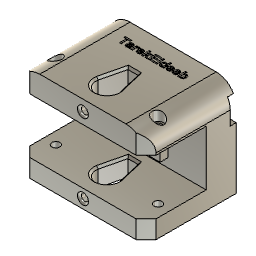
pltr_base_elegoo (Autodesk Fusion 360 design; units mm, degrees)
Autodesk Fusion 360 part; units mm, degrees
sketch "Top" plane through (0, 0, 0) normal (0, 0, 1) x (1, 0, 0)
  line L0 (0, 0) -> (-63, 0)
  line L1 (-63, 0) -> (-63, 35)
  line L2 (-63, 35) -> (0, 35)
  line L3 (0, 35) -> (0, 0)
  line L4 (-63, 12) -> (0, 12)
  line L5 (-6, 35) -> (-6, 0)
  line L6 (-57, 0) -> (-57, 35)
  line L7 (-31.5, 35) -> (-31.5, 0)
  line L8 (-63, 25) -> (0, 25)
  circle A0 centre (-31.5, 12) radius 5.5
  line L9 (-34, 25) -> (-29, 25)
  line L10 (-34, 25) -> (-36.91568, 12.95938)
  line L11 (-29, 25) -> (-26.15564, 13.299162)
  circle A1 centre (-6, 12) radius 3
  circle A2 centre (-6, 12) radius 2
  circle A3 centre (-57, 12) radius 3
  circle A4 centre (-57, 12) radius 2
  line L12 (-63, 35) -> (0, 35)
  line L13 (0, 35) -> (0, 45)
  line L14 (0, 45) -> (-63, 45)
  line L15 (-63, 45) -> (-63, 35)
  line L16 (-3.293913, 9.66023) -> (-2.620656, 13.173655)
  line L17 (-2.620656, 13.173655) -> (-5.326743, 15.513426)
  line L18 (-5.326743, 15.513426) -> (-8.706088, 14.339771)
  line L19 (-8.706088, 14.339771) -> (-9.379345, 10.826345)
  line L20 (-9.379345, 10.826345) -> (-6.673257, 8.486574)
  line L21 (-6.673257, 8.486574) -> (-3.293913, 9.66023)
  line L22 (-57.673257, 15.513426) -> (-54.293912, 14.339771)
  line L23 (-54.293912, 14.339771) -> (-53.620655, 10.826345)
  line L24 (-53.620655, 10.826345) -> (-56.326743, 8.486574)
  line L25 (-56.326743, 8.486574) -> (-59.706087, 9.66023)
  line L26 (-60.379344, 13.173655) -> (-57.673257, 15.513426)
  line L27 (-59.706087, 9.66023) -> (-60.379344, 13.173655)
  point P0 (-6, 12)
  dimension "d1" = 35
  dimension "d2" = 63
  dimension "d3" = 12
  dimension "d4" = 6
  dimension "d5" = 6
  dimension "d6" = 31.5
  dimension "d7" = 10
  dimension "d8" = 11
  dimension "d9" = 5
  dimension "d10" = 6
  dimension "d11" = 4
  dimension "d30" = 10
  constraint horizontal L0
  constraint vertical L1
  constraint horizontal L2
  constraint vertical L3
  constraint coincident L0.start L3.end
  constraint coincident L1 L4.start
  constraint coincident L3 L4.end
  constraint perpendicular L3 L4
  constraint coincident L2 L5.start
  constraint coincident L0 L5.end
  constraint perpendicular L0 L5
  constraint coincident L0 L6.start
  constraint coincident L2 L6.end
  constraint perpendicular L2 L6
  constraint coincident L2 L7.start
  constraint coincident L0 L7.end
  constraint perpendicular L0 L7
  constraint coincident L1 L8.start
  constraint coincident L3 L8.end
  constraint perpendicular L3 L8
  constraint midpoint L4 A0.centre
  constraint coincident L8 L9.start
  constraint coincident L8 L9.end
  constraint midpoint L8 L9
  constraint tangent A0 L11
  constraint coincident L5 P0
  constraint coincident L4 P0
  constraint concentric A1 A2
  constraint symmetric L7 A1 A3
  constraint symmetric L7 A2 A4
  constraint coincident P0 A1.centre
  constraint horizontal L12
  constraint vertical L13
  constraint horizontal L14
  constraint vertical L15
  constraint collinear L3 L13
  measures "d1" distance of L0.start L2.end
  measures "d2" distance of L0.start L0.end
  measures "d3" distance of L0 L4
  measures "d4" distance of L3 L5
  measures "d5" distance of L1 L6
  measures "d6" distance of L1 L7
  measures "d7" distance of L2 L8
  measures "d8" diameter of A0
  measures "d9" distance of L9.start L9.end
  measures "d10" diameter of A1
  measures "d11" diameter of A2
  measures "d30" distance of L12 L14
extrude "Extrude1" add sketch "Top" along normal blind 47.5 contours L0 L3 L4 L5 L16 L21 | L0 L4 L5 L7 A0 L19 L20 L21 | L3 L4 L5 L8 L16 L17 L18 | L0 L4 L6 L7 A0 L23 L24 L25 | L4 L5 A1 L19 L20 L21 | L4 L5 A1 L16 L21 | L2 L3 L5 L8 L12 | L4 L5 A1 L16 L17 L18 | L0 L1 L4 L6 L25 L27 | L4 L7 A0 | L4 L7 A0 | L4 L5 A1 A2 | L4 L5 A1 A2 | L2 L12 L13 L14 L15 | L2 L5 L7 L8 L9 L12 | L4 L5 L8 A0 L11 L18 L19 | L4 L5 A1 A2 | L4 L6 A3 L25 L27 | L4 L6 A3 L23 L24 L25 | L4 L7 A0 | L4 L7 A0 L10 | L4 L6 L8 A0 L10 L22 L23 | L4 L5 A2 | L4 L5 A2 | L4 L5 A1 A2 | L4 L5 A1 L18 L19 | L7 L8 A0 L9 L11 | L4 L5 A2 | L1 L4 L6 L8 L22 L26 L27 | L4 L6 A3 A4 | L4 L6 A3 A4 | L7 L8 A0 L9 L10 | L4 L6 A3 L22 L23 | A0 L10 | L4 L5 A2 | L2 L6 L7 L8 L9 L12 | L1 L2 L6 L8 L12 | L4 L6 A3 L22 L26 L27 | L4 L6 A4 | L4 L6 A4 | L4 L6 A3 A4 | L4 L6 A3 A4 | L4 L6 A4 | L4 L6 A4 picked at (-4, 2.906799) picked at (-14.08415, 6.617607) picked at (-3.775581, 21.837809) picked at (-48.91585, 6.617607) picked at (-6.366734, 8.745836) picked at (-3.500968, 10.024575) picked at (-4, 31.666667) picked at (-5.633266, 15.254164) picked at (-59, 2.906799) picked at (-34.086119, 9.413881) picked at (-27.851994, 11.739089) picked at (-8.656488, 11.857685) picked at (-5.857685, 9.343512) picked at (-31.5, 41.666667) picked at (-22.166667, 31.666667) picked at (-14.568696, 21.44659) picked at (-5.857685, 14.656488) picked at (-59.499032, 10.024575) picked at (-56.633266, 8.745836) picked at (-28.84098, 14.510086) picked at (-34.909433, 13.324121) picked at (-48.431304, 21.44659) picked at (-7.326548, 11.905123) picked at (-4.673452, 11.905124) picked at (-8.649703, 12.237191) picked at (-8.499032, 13.975425) picked at (-30.396256, 22.479948) picked at (-5.905123, 13.326548) picked at (-59.224419, 21.837809) picked at (-59.656488, 11.857685) picked at (-56.762809, 9.350298) picked at (-32.591374, 22.48175) picked at (-54.500968, 13.975425) picked at (-36.829268, 13.32964) picked at (-6.637371, 13.167257) picked at (-40.833333, 31.666667) picked at (-61, 31.666667) picked at (-57.366734, 15.254164) picked at (-58.326548, 11.905123) picked at (-55.673452, 11.905124) picked at (-59.649702, 12.237191) picked at (-56.762809, 14.649703) picked at (-56.362629, 13.167257) picked at (-57.094877, 13.326548)
sketch "Front" plane through (0, 0, 0) normal (0, 1, 0) x (1, 0, 0)
  line L0 (0, 0) -> (-73.000001, 0)
  line L1 (0, 0) -> (0, -54.383699)
  line L2 (0, -9) -> (-63.000001, -9)
  line L3 (0, -36.5) -> (-63.000001, -36.5)
  line L4 (-63, -47.5) -> (0, -47.5)
  line L5 (0, 0) -> (-63, 0)
  line L6 (-31.5, 0) -> (-31.5, -47.5)
  circle A0 centre (-31.5, -42) radius 1.75
  circle A1 centre (-31.5, -4.5) radius 1.75
  line L7 (0, -32) -> (-63.000001, -32)
  circle A2 centre (-23.75, -32) radius 3.5
  line L8 (-20.615874, -33.729332) -> (-20.685292, -30.150433)
  line L9 (-20.685292, -30.150433) -> (-23.819418, -28.421101)
  line L10 (-23.819418, -28.421101) -> (-26.884126, -30.270668)
  line L11 (-26.884126, -30.270668) -> (-26.814708, -33.849567)
  line L12 (-26.814708, -33.849567) -> (-23.680582, -35.578899)
  line L13 (-23.680582, -35.578899) -> (-20.615874, -33.729332)
  circle A3 centre (-39.25, -32) radius 3.5
  line L14 (-39.319418, -35.578899) -> (-42.384126, -33.729332)
  line L15 (-36.185292, -33.849567) -> (-39.319418, -35.578899)
  line L16 (-36.115874, -30.270668) -> (-36.185292, -33.849567)
  line L17 (-39.180582, -28.421101) -> (-36.115874, -30.270668)
  line L18 (-42.314708, -30.150433) -> (-39.180582, -28.421101)
  line L19 (-42.384126, -33.729332) -> (-42.314708, -30.150433)
  circle A4 centre (-31.5, -5) radius 3.5
  line L20 (-1, -47.5) -> (-1, 0)
  circle A5 centre (-1, -36.5) radius 6
  circle A6 centre (-62, -36.5) radius 6
  line L21 (-63, 0) -> (-63, -47.5)
  line L22 (-19, -9) -> (-19, -32)
  line L23 (-19, -23.444466) -> (-24.5, -23.444466)
  line L24 (-24.5, -23.444466) -> (-24.5, -13.444466)
  line L25 (-24.5, -13.444466) -> (-19, -13.444466)
  line L26 (-19, -13.444466) -> (-19, -23.444466)
  line L27 (-67.000001, 2) -> (5, 2)
  line L28 (-63.000001, -9) -> (-63, 0)
  line L29 (0, 0) -> (0, 9)
  circle A7 centre (-16, 2) radius 6
  circle A8 centre (-47, 2) radius 6
  circle A9 centre (-23.75, -32) radius 1.75
  circle A10 centre (-39.25, -32) radius 1.75
  point P0 (-23.75, -32)
  dimension "d14" = 9
  dimension "d15" = 11
  dimension "d16" = 3.5
  dimension "d17" = 5.5
  dimension "d18" = 3.5
  dimension "d19" = 4.5
  dimension "d20" = 32
  dimension "d22" = 7.75
  dimension "d23" = 7
  dimension "d24" = 3.1
  dimension "d25" = 7
  dimension "d26" = 5
  dimension "d27" = 1
  dimension "d28" = 12
  dimension "d29" = 11
  dimension "d61" = 19
  dimension "d62" = 5.5
  dimension "d63" = 10
  dimension "d67" = 2
  dimension "d68" = 12
  dimension "d69" = 16
  dimension "d72" = 3.5
  dimension "d73" = 3.5
  constraint coincident L0.start L1.start
  constraint horizontal L0
  constraint perpendicular L0 L1
  constraint coincident L1 L2.start
  constraint perpendicular L1 L2
  constraint coincident L1 L3.start
  constraint perpendicular L1 L3
  constraint midpoint L5 L6.start
  constraint midpoint L4 L6.end
  constraint coincident L6 A0.centre
  constraint coincident L6 A1.centre
  constraint coincident L1 L7.start
  constraint perpendicular L1 L7
  constraint coincident P0 A2.centre
  constraint symmetric L6 A2 A3
  constraint coincident L6 A4.centre
  constraint coincident L4 L20.start
  constraint coincident L0 L20.end
  constraint perpendicular L0 L20
  constraint coincident L20 A5.centre
  constraint symmetric L6 A5 A6
  constraint coincident L5.end L21.start
  constraint coincident L4.start L21.end
  constraint coincident L2 L22.start
  constraint coincident L7 L22.end
  constraint perpendicular L7 L22
  constraint horizontal L23
  constraint vertical L24
  constraint horizontal L25
  constraint vertical L26
  constraint horizontal L27
  constraint perpendicular L27 L29
  constraint coincident L27 A7.centre
  constraint symmetric L6 A7 A8
  constraint concentric A2 A9
  constraint concentric A3 A10
  measures "d14" distance of L0 L2
  measures "d15" distance of L3 L4
  measures "d16" diameter of A0
  measures "d17" distance of L4 A0.centre
  measures "d18" diameter of A1
  measures "d19" distance of L0 A1.centre
  measures "d20" distance of L0 L7
  measures "d22" distance of L6 P0
  measures "d24" distance of P0 L13
  measures "d25" diameter of A4
  measures "d26" distance of L6.start A4.centre
  measures "d27" distance of L1 L20
  measures "d28" diameter of A5
  measures "d29" distance of L4 A5.centre
  measures "d61" distance of L1 L22
  measures "d67" distance of L0 L27
  measures "d68" diameter of A7
  measures "d69" distance of L29 A7.centre
  measures "d73" diameter of A10
extrude "Extrude2" cut sketch "Front" along normal blind 30 contours L1 L2 L20 A5 | L2 L7 L20 A5 L22 L26 | L1 L7 L20 A5 | L2 L6 L7 A2 L8 L9 L10 L11 L22 L23 L24 L25 | L7 L20 A5 | L1 L3 L7 L20 | L2 L6 L7 A3 L16 L17 L18 L19 A6 L21 | L22 L23 L24 L25 L26 | L3 L7 L20 A5 | L3 L6 L7 A2 L8 L11 L12 L13 A5 | L3 L6 L7 A3 L14 L15 L16 L19 A6 | L7 A6 L21 | L7 A2 L11 | L7 A2 L11 | L7 A3 L16 | L7 A3 L16 | L7 A2 L8 | L7 A2 L8 | L3 L7 A6 L21 | L7 A2 L8 L9 L10 L11 A9 | L7 A2 L8 L11 L12 L13 A9 | A2 L10 L11 | A2 L11 L12 | L7 A3 L14 L15 L16 L19 A10 | L7 A3 L16 L17 L18 L19 A10 | A3 L16 L17 | A3 L15 L16 | A2 L8 L9 | A2 L8 L13 | L7 A3 L19 | L7 A3 L19 | L7 A9 | L7 A9 | A2 L10 | A2 L12 | L7 A10 | L7 A10 | A3 L17 | A3 L15 | A2 L9 | A2 L13 | A3 L18 L19 | A3 L14 L19 | A2 L9 L10 | A2 L12 L13 | A3 L17 L18 | A3 L14 L15 | A3 L18 | A3 L14 picked at (-0.555093, -16.169781) picked at (-7.570167, -21.064483) picked at (-0.443866, -31.512449) picked at (-29.166667, -21.481489) picked at (-1.288088, -31.020857) picked at (-0.666667, -33.5) picked at (-45.075231, -15.608769) picked at (-22.666667, -16.7778) picked at (-2.322876, -33.5) picked at (-30.001565, -33.929076) picked at (-32.998435, -33.929076) picked at (-62.704833, -31.028338) picked at (-27.109042, -31.865152) picked at (-27.10768, -32.146079) picked at (-35.89232, -32.146079) picked at (-35.890958, -31.865152) picked at (-20.390958, -32.134848) picked at (-20.39232, -31.853921) picked at (-61.343791, -33.5) picked at (-25.109515, -29.725408) picked at (-25.040097, -34.31467) picked at (-26.83749, -30.296401) picked at (-26.769105, -33.822045) picked at (-37.959903, -34.31467) picked at (-40.540097, -29.68533) picked at (-36.16251, -30.296401) picked at (-36.230895, -33.822045) picked at (-20.730895, -30.177955) picked at (-20.66251, -33.703599) picked at (-42.60768, -31.853921) picked at (-42.609042, -32.134848) picked at (-23.706407, -31.418298) picked at (-24.294966, -32.511981) picked at (-25.613001, -29.376867) picked at (-25.624183, -34.580312) picked at (-39.807417, -32.171941) picked at (-39.541667, -30.837612) picked at (-37.649601, -29.192563) picked at (-37.375817, -34.580312) picked at (-22.099535, -29.147131) picked at (-22.452476, -34.913246) picked at (-42.269105, -30.177955) picked at (-42.33749, -33.703599) picked at (-23.818385, -28.474355) picked at (-23.681615, -35.525645) picked at (-39.181615, -28.474355) picked at (-39.318385, -35.525645) picked at (-40.783445, -29.082562) picked at (-41.222833, -34.505694)
extrude "Extrude3" cut sketch "Top" along normal blind 65 contours L4 L7 A0 | L4 L7 A0 | L4 L7 A0 | L4 L7 A0 L10 | L7 L8 A0 L9 L11 | L7 L8 A0 L9 L10 picked at (-34.086119, 9.413881) picked at (-27.851994, 11.739089) picked at (-28.84098, 14.510086) picked at (-34.909433, 13.324121) picked at (-30.396256, 22.479948) picked at (-32.591374, 22.48175)
extrude "Extrude4" cut sketch "Top" along normal blind 6 from surface at 42.5 contours L4 L5 A1 A2 | L4 L5 A1 A2 | L4 L5 A1 A2 | L4 L5 A2 | L4 L5 A2 | L4 L5 A1 A2 | L4 L5 A2 | L4 L6 A3 A4 | L4 L6 A3 A4 | L4 L5 A2 | L4 L6 A4 | L4 L6 A4 | L4 L6 A3 A4 | L4 L6 A3 A4 | L4 L6 A4 | L4 L6 A4 picked at (-8.656488, 11.857685) picked at (-5.857685, 9.343512) picked at (-5.857685, 14.656488) picked at (-7.326548, 11.905123) picked at (-4.673452, 11.905124) picked at (-8.649703, 12.237191) picked at (-5.905123, 13.326548) picked at (-59.656488, 11.857685) picked at (-56.762809, 9.350298) picked at (-6.637371, 13.167257) picked at (-58.326548, 11.905123) picked at (-55.673452, 11.905124) picked at (-59.649702, 12.237191) picked at (-56.762809, 14.649703) picked at (-56.362629, 13.167257) picked at (-57.094877, 13.326548)
extrude "Extrude5" cut sketch "Top" along normal blind 47.5 contours L4 L5 A2 | L4 L5 A2 | L4 L5 A2 | L4 L5 A2 | L4 L6 A4 | L4 L6 A4 | L4 L6 A4 | L4 L6 A4 picked at (-7.326548, 11.905123) picked at (-4.673452, 11.905124) picked at (-5.905123, 13.326548) picked at (-6.637371, 13.167257) picked at (-58.326548, 11.905123) picked at (-55.673452, 11.905124) picked at (-56.362629, 13.167257) picked at (-57.094877, 13.326548)
extrude "Extrude6" cut sketch "Top" along normal blind 5 contours L4 L5 A1 L19 L20 L21 | L4 L5 A1 L16 L21 | L4 L5 A1 L16 L17 L18 | L4 L5 A1 A2 | L4 L5 A1 A2 | L4 L5 A1 A2 | L4 L6 A3 L25 L27 | L4 L6 A3 L23 L24 L25 | L4 L5 A1 A2 | L4 L5 A1 L18 L19 | L4 L6 A3 A4 | L4 L6 A3 A4 | L4 L6 A3 L22 L23 | L4 L6 A3 L22 L26 L27 | L4 L6 A3 A4 | L4 L6 A3 A4 picked at (-6.366734, 8.745836) picked at (-3.500968, 10.024575) picked at (-5.633266, 15.254164) picked at (-8.656488, 11.857685) picked at (-5.857685, 9.343512) picked at (-5.857685, 14.656488) picked at (-59.499032, 10.024575) picked at (-56.633266, 8.745836) picked at (-8.649703, 12.237191) picked at (-8.499032, 13.975425) picked at (-59.656488, 11.857685) picked at (-56.762809, 9.350298) picked at (-54.500968, 13.975425) picked at (-57.366734, 15.254164) picked at (-59.649702, 12.237191) picked at (-56.762809, 14.649703)
chamfer "Chamfer1" distance 5 angle 45 4 edges at (0, 0, 42) (-63, 0, 42) (-63, 0, 4.5) (0, 0, 4.5)
fillet "Fillet1" radius 10 2 edges at (0, 25, 47.5) (-63, 25, 47.5)
chamfer "Chamfer2" distance 1 angle 45 8 edges at (-35.45784, 18.97969, 47.5) (-31.326407, 6.50274, 47.5) (-27.57782, 19.149581, 47.5) (-31.5, 25, 47.5) (-35.45784, 18.97969, 9) (-31.326407, 6.50274, 9) (-27.57782, 19.149581, 9) (-31.5, 25, 9)
extrude "Extrude7" cut sketch "Front" along normal blind 10 contours L6 A1 | L6 A1 | L6 A0 | L6 A0 picked at (-30.940296, -4.335656) picked at (-32.537771, -4.092705) picked at (-30.730458, -41.617998) picked at (-32.537771, -41.592705)
fillet "Fillet2" radius 1 2 edges at (-33.131573, 0, 42.632827) (-33.131573, 0, 5.132827)
extrude "Extrude8" cut sketch "Front" along normal blind 33 contours L7 A2 L8 L9 L10 L11 A9 | L7 A2 L8 L11 L12 L13 A9 | A2 L10 L11 | A2 L11 L12 | L7 A3 L14 L15 L16 L19 A10 | L7 A3 L16 L17 L18 L19 A10 | A3 L16 L17 | A3 L15 L16 | A2 L8 L9 | A2 L8 L13 | L7 A9 | L7 A9 | L7 A10 | L7 A10 | A3 L18 L19 | A3 L14 L19 | A2 L9 L10 | A2 L12 L13 | A3 L17 L18 | A3 L14 L15 picked at (-25.109515, -29.725408) picked at (-25.040097, -34.31467) picked at (-26.83749, -30.296401) picked at (-26.769105, -33.822045) picked at (-37.959903, -34.31467) picked at (-40.540097, -29.68533) picked at (-36.16251, -30.296401) picked at (-36.230895, -33.822045) picked at (-20.730895, -30.177955) picked at (-20.66251, -33.703599) picked at (-23.706407, -31.418298) picked at (-24.294966, -32.511981) picked at (-39.807417, -32.171941) picked at (-39.541667, -30.837612) picked at (-42.269105, -30.177955) picked at (-42.33749, -33.703599) picked at (-23.818385, -28.474355) picked at (-23.681615, -35.525645) picked at (-39.181615, -28.474355) picked at (-39.318385, -35.525645)
extrude "Extrude9" cut sketch "Front" along normal blind 8 from surface at 37 contours L7 A2 L11 | L7 A2 L11 | L7 A3 L16 | L7 A3 L16 | L7 A2 L8 | L7 A2 L8 | L7 A2 L8 L9 L10 L11 A9 | L7 A2 L8 L11 L12 L13 A9 | L7 A3 L14 L15 L16 L19 A10 | L7 A3 L16 L17 L18 L19 A10 | L7 A3 L19 | L7 A3 L19 | L7 A9 | L7 A9 | A2 L10 | A2 L12 | L7 A10 | L7 A10 | A3 L17 | A3 L15 | A2 L9 | A2 L13 | A3 L18 | A3 L14 picked at (-27.109042, -31.865152) picked at (-27.10768, -32.146079) picked at (-35.89232, -32.146079) picked at (-35.890958, -31.865152) picked at (-20.390958, -32.134848) picked at (-20.39232, -31.853921) picked at (-25.109515, -29.725408) picked at (-25.040097, -34.31467) picked at (-37.959903, -34.31467) picked at (-40.540097, -29.68533) picked at (-42.60768, -31.853921) picked at (-42.609042, -32.134848) picked at (-23.706407, -31.418298) picked at (-24.294966, -32.511981) picked at (-25.613001, -29.376867) picked at (-25.624183, -34.580312) picked at (-39.807417, -32.171941) picked at (-39.541667, -30.837612) picked at (-37.649601, -29.192563) picked at (-37.375817, -34.580312) picked at (-22.099535, -29.147131) picked at (-22.452476, -34.913246) picked at (-40.783445, -29.082562) picked at (-41.222833, -34.505694)
extrude "Extrude10" cut sketch "Front" along normal blind 10 from surface at 35 contours L6 A1 A4 | L6 A1 A4 | L6 A1 | L6 A1 picked at (-30.922261, -7.684929) picked at (-32.104705, -7.678622) picked at (-30.940296, -4.335656) picked at (-32.537771, -4.092705)
extrude "Extrude11" cut sketch "Front" along normal blind 5 from surface at 42 contours L0 L5 A7 | L1 L7 L20 A5 | L7 L20 A5 | L1 L3 L7 L20 | L3 L7 L20 A5 | L1 L3 L20 A5 | L0 L5 A8 | L3 L20 A5 | L7 A6 L21 | L3 L7 A6 L21 | L3 A6 L21 picked at (-17.213053, -0.92346) picked at (-0.443866, -31.512449) picked at (-1.288088, -31.020857) picked at (-0.666667, -33.5) picked at (-2.322876, -33.5) picked at (-0.333333, -38.472027) picked at (-45.518003, -1.434233) picked at (-4.979643, -36.78463) picked at (-62.704833, -31.028338) picked at (-61.343791, -33.5) picked at (-58.35428, -36.788695)
extrude "Extrude12" add sketch "Front" along normal blind 4 from surface at 26 contours L22 L23 L24 L25 L26 picked at (-22.666667, -16.7778)
extrude "Extrude13" cut sketch "Front" along normal blind 45 contours L7 A9 | L7 A9 | L7 A10 | L7 A10 picked at (-23.706407, -31.418298) picked at (-24.294966, -32.511981) picked at (-39.807417, -32.171941) picked at (-39.541667, -30.837612)
ref_plane "WorkPlane1" through (-31.5, 22.5, 47.5) normal (0, 0, 1) x (1, 0, 0)
sketch "Sketch3" plane through (0, 0, 47.5) normal (0, 0, 1) x (1, 0, 0)
  line L0 (-47.913005, 28.563237) -> (-13.913005, 28.563237) construction
  line L1 (-13.913005, 28.563237) -> (-13.913005, 37.563237) construction
  line L2 (-13.913005, 37.563237) -> (-47.913005, 37.563237) construction
  line L3 (-47.913005, 37.563237) -> (-47.913005, 28.563237) construction
  dimension "d77" = 4
  text T0 "TarekEldeeb" font "Arial" height 4 bold align left top in box 34.000001 x 9 at (-47.913005, 28.563237) x (1, 0) y (0, 1) spacing 1
extrude "Extrude15" cut sketch "Sketch3" against normal blind 0.7 text T0
